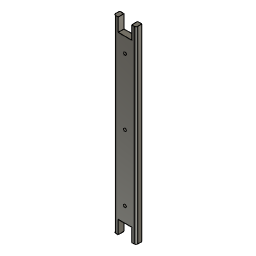
Y_Extrusion_Positioner v4 (Autodesk Fusion 360 design; units mm, degrees)
Autodesk Fusion 360 part; units mm, degrees
sketch "Sketch1" plane through (0, 0, 0) normal (0, 1, 0) x (1, 0, 0)
  line L0 (7.6, 7.5) -> (-7.6, 7.5)
  line L1 (-7.6, 7.5) -> (-7.6, -7.5)
  line L2 (-7.6, -7.5) -> (7.6, -7.5)
  line L3 (7.6, -7.5) -> (7.6, 7.5)
  line L4 (7.6, 7.5) -> (-7.6, -7.5) construction
  line L5 (-7.6, 7.5) -> (7.6, -7.5) construction
  line L6 (7.6, -192) -> (-7.6, -192)
  line L7 (-7.6, -192) -> (-7.6, -207)
  line L8 (-7.6, -207) -> (7.6, -207)
  line L9 (7.6, -207) -> (7.6, -192)
  line L10 (7.6, -192) -> (-7.6, -207) construction
  line L11 (-7.6, -192) -> (7.6, -207) construction
  circle A0 centre (0, -174.75) radius 1.6
  circle A1 centre (0, -99.75) radius 1.6
  circle A2 centre (0, -24.75) radius 1.6
  line L12 (12.6, -207) -> (-12.6, -207)
  line L13 (-12.6, -207) -> (-12.6, 7.5)
  line L14 (-12.6, 7.5) -> (12.6, 7.5)
  line L15 (12.6, 7.5) -> (12.6, -207)
  line L16 (12.6, -207) -> (-12.6, 7.5) construction
  line L17 (-12.6, -207) -> (12.6, 7.5) construction
  point P0 (0, -199.5)
  point P1 (0, -99.75)
  dimension "d1" = 15.2
  dimension "d2" = 15
  dimension "d3" = 15.2
  dimension "d4" = 15
  dimension "d5" = 184.5
  dimension "d6" = 3.2
  dimension "d12" = 0
  dimension "d13" = 150
  dimension "d14" = 25.2
  dimension "d20" = 207
  constraint horizontal L0
  constraint perpendicular L0 L1
  constraint parallel L0 L2
  constraint parallel L1 L3
  constraint coincident L4 origin
  constraint coincident L5 origin
  constraint horizontal L6
  constraint perpendicular L6 L7
  constraint parallel L6 L8
  constraint parallel L7 L9
  constraint coincident L10 P0
  constraint coincident L11 P0
  constraint vertical origin P0
  constraint vertical origin A2.centre
  constraint horizontal L12
  constraint perpendicular L12 L13
  constraint parallel L12 L14
  constraint parallel L13 L15
  constraint coincident L16 P1
  constraint coincident L17 P1
  constraint coincident P1 A1.centre
  constraint horizontal L7.end L12.end
  constraint horizontal L0.end L13.end
  measures "d1" distance of L1.end L2.end
  measures "d2" distance of L0.end L1.end
  measures "d3" distance of L7.end L8.end
  measures "d4" distance of L6.end L7.end
  measures "d5" distance of L2 L6
  measures "d6" diameter of A0
  measures "d14" distance of L12.start L12.end
  measures "d20" vertical distance of P0 L14.end
extrude "Extrude1" add sketch "Sketch1" along normal blind 7 contours L1 L2 L3 L6 L7 L9 L12 L13 L14 L15
fillet "Fillet1" radius 2 2 edges at (-12.6, 0, 99.75) (12.6, 0, 99.75)
move_face "OffsetFaces1" offset -0.1 3 faces at (-7.6, 2.3333, 197) (7.6, 2.3333, 202) (2.5333, 2.3333, 192)
move_face "OffsetFaces2" offset -0.1 3 faces at (-2.5333, 2.3333, 7.5) (-7.6, 2.3333, -2.5) (7.6, 2.3333, 2.5)
chamfer "Chamfer1" distance 0.4 angle 45 1 faces at (0, 7, 12.7833)
equation "d14 = 15.2 mm + 10 mm"
named bodies: "y_extusion_positioner"
